J13 (Autodesk Fusion 360 design; units mm, degrees)
part number: 2026-05-31-16-59-09-966
Autodesk Fusion 360 part; units mm, degrees
sketch "Sketch1" plane through (0, 0, 0) normal (0, 0, 1) x (1, 0, 0)
  line L0 (0, 0) -> (40, 0)
  line L1 (40, 0) -> (40, 40)
  line L2 (40, 40) -> (0, 40)
  line L3 (0, 40) -> (0, 0)
  dimension "d1" = 40
  dimension "d2" = 40
  constraint horizontal L0
  constraint vertical L1
  constraint horizontal L2
  constraint vertical L3
  constraint coincident L0.start L3.end
  measures "d1" distance of L0.start L0.end
  measures "d2" distance of L0.start L2.end
extrude "Extrude1" add sketch "Sketch1" along normal blind 5 makes body 1
sketch "Sketch2" plane through (0, 0, 5) normal (0, 0, 1) x (-1, 0, 0)
  line L0 (0, -40) -> (0, 0)
  line L1 (0, 0) -> (-40, 0)
  line L2 (-40, 0) -> (-40, -40)
  line L3 (-40, -40) -> (0, -40)
  line L4 (0, -40) -> (-40, -40)
  line L5 (-40, -40) -> (-40, 0)
  line L6 (-40, 0) -> (0, 0)
  line L7 (0, 0) -> (0, -40)
  line L8 (-38.5, -1.5) -> (-1.5, -1.5)
  line L9 (-1.5, -1.5) -> (-1.5, -38.5)
  line L10 (-1.5, -38.5) -> (-38.5, -38.5)
  line L11 (-38.5, -38.5) -> (-38.5, -1.5)
  constraint horizontal L4
  constraint vertical L5
  constraint horizontal L6
  constraint vertical L7
  constraint coincident L1.end L2.start
  constraint coincident L0.start L3.end
  constraint horizontal L8
  constraint vertical L9
  constraint horizontal L10
  constraint vertical L11
extrude "Extrude2" add sketch "Sketch2" along normal blind 30 bodies 1
sketch "Sketch3" plane through (0, 0, 5) normal (0, 0, 1) x (-1, 0, 0)
  line L0 (-1.5, -38.5) -> (-1.5, -1.5)
  line L1 (-1.5, -1.5) -> (-38.5, -1.5)
  line L2 (-38.5, -1.5) -> (-38.5, -38.5)
  line L3 (-38.5, -38.5) -> (-1.5, -38.5)
  circle A0 centre (-20, -20) radius 15.2
  dimension "d7" = 30.4
  measures "d7" diameter of A0
extrude "Extrude3" cut sketch "Sketch3" against normal blind 49 contours A0 bodies 1
sketch "Sketch4" plane through (0, 0, 0) normal (0, 0, -1) x (1, 0, 0)
  circle A0 centre (20, -20) radius 15.2
  line L0 (0, 0) -> (0, -40)
  line L1 (0, -40) -> (40, -40)
  line L2 (40, -40) -> (40, 0)
  line L3 (40, 0) -> (0, 0)
  circle A1 centre (20, -20) radius 18.2
  dimension "d10" = 3
extrude "Extrude4" add sketch "Sketch4" along normal blind 25 contours A1 bodies 1
sketch "Sketch5" plane through (0, 0, 0) normal (-1, 0, 0) x (0, -1, 0)
  line L0 (-40, 0) -> (0, 0)
  line L1 (0, 0) -> (0, 35)
  line L2 (0, 35) -> (-40, 35)
  line L3 (-40, 35) -> (-40, 0)
  circle A0 centre (-20, -20) radius 1.25
  circle A1 centre (-20, -8) radius 1.25
  dimension "d13" = 2.5
  dimension "d14" = 2.5
  measures "d13" diameter of A0
  measures "d14" diameter of A1
extrude "Extrude5" cut sketch "Sketch5" against normal blind 49 contours A0 | A1 bodies 1
sketch "Sketch6" plane through (0, 0, 0) normal (-1, 0, 0) x (0, -1, 0)
  line L0 (-40, 0) -> (0, 0)
  line L1 (0, 0) -> (0, 35)
  line L2 (0, 35) -> (-40, 35)
  line L3 (-40, 35) -> (-40, 0)
extrude "Extrude6" add sketch "Sketch6" along normal blind 10 bodies 1
sketch "Sketch7" plane through (1.5, 0, 0) normal (1, 0, 0) x (0, 1, 0)
  line L0 (1.5, 5) -> (38.5, 5)
  line L1 (38.5, 5) -> (38.5, 35)
  line L2 (38.5, 35) -> (1.5, 35)
  line L3 (1.5, 35) -> (1.5, 5)
  line L4 (3.5, 7) -> (36.5, 7)
  line L5 (36.5, 7) -> (36.5, 33)
  line L6 (36.5, 33) -> (3.5, 33)
  line L7 (3.5, 33) -> (3.5, 7)
  dimension "d19" = -2
extrude "Extrude7" cut sketch "Sketch7" against normal blind 10 contours L4 L5 L6 L7 bodies 1
fillet "Fillet1" radius 5 1 faces at (-10, 26.6667, 23.3333) on bodies 1
sketch "Sketch8" plane through (38.5, 0, 0) normal (-1, 0, 0) x (0, -1, 0)
  line L0 (-38.5, 5) -> (-1.5, 5)
  line L1 (-1.5, 5) -> (-1.5, 35)
  line L2 (-1.5, 35) -> (-38.5, 35)
  line L3 (-38.5, 35) -> (-38.5, 5)
extrude "Extrude8" cut sketch "Sketch8" against normal blind 7 bodies 1
sketch "Sketch9" plane through (40, 0, 0) normal (1, 0, 0) x (0, 1, 0)
  line L0 (38.5, 35) -> (38.5, 5)
  line L1 (38.5, 5) -> (1.5, 5)
  line L2 (1.5, 5) -> (1.5, 35)
  line L3 (1.5, 35) -> (0, 35)
  line L4 (0, 35) -> (0, 0)
  line L5 (0, 0) -> (40, 0)
  line L6 (40, 0) -> (40, 35)
  line L7 (40, 35) -> (38.5, 35)
  line L8 (0, 35) -> (1.5, 35)
  line L9 (1.5, 35) -> (1.5, 0)
  line L10 (1.5, 0) -> (0, 0)
  line L11 (0, 0) -> (0, 35)
  constraint horizontal L8
  constraint vertical L9
  constraint horizontal L10
  constraint vertical L11
  constraint coincident L5 L9.end
  constraint coincident L3.end L4.start
extrude "Extrude9" add sketch "Sketch9" along normal blind 24 contours L2 L3 L4 L5 L8 L9 L10 L11 bodies 1
sketch "Sketch10" plane through (0, 1.5, 0) normal (0, 1, 0) x (-1, 0, 0)
  line L0 (-40, 5) -> (-1.5, 5)
  line L1 (-1.5, 5) -> (-1.5, 35)
  line L2 (-1.5, 35) -> (-64, 35)
  line L3 (-64, 35) -> (-64, 0)
  line L4 (-64, 0) -> (-40, 0)
  line L5 (-40, 0) -> (-40, 5)
  line L6 (-64, 35) -> (-60, 35)
  line L7 (-60, 35) -> (-60, 0)
  line L8 (-60, 0) -> (-64, 0)
  line L9 (-64, 0) -> (-64, 35)
  constraint horizontal L6
  constraint vertical L7
  constraint horizontal L8
  constraint vertical L9
  constraint coincident L4 L7.end
  constraint coincident L2.end L3.start
extrude "Extrude10" add sketch "Sketch10" along normal blind 40 contours L2 L3 L4 L6 L7 L8 L9 bodies 1
sketch "Sketch11" plane through (60, 0, 0) normal (-1, 0, 0) x (0, -1, 0)
  line L0 (-1.5, 0) -> (-1.5, 35)
  line L1 (-1.5, 35) -> (-41.5, 35)
  line L2 (-41.5, 35) -> (-41.5, 0)
  line L3 (-41.5, 0) -> (-1.5, 0)
  line L4 (-41.5, 35) -> (-35, 35)
  line L5 (-35, 35) -> (-35, 0)
  line L6 (-35, 0) -> (-41.5, 0)
  line L7 (-41.5, 0) -> (-41.5, 35)
  constraint horizontal L4
  constraint vertical L5
  constraint horizontal L6
  constraint vertical L7
  constraint coincident L3 L5.end
  constraint coincident L1.end L2.start
extrude "Extrude11" add sketch "Sketch11" along normal blind 7 contours L1 L2 L3 L4 L5 L6 L7 bodies 1
sketch "Sketch12" plane through (40, 0, 0) normal (1, 0, 0) x (0, 1, 0)
  line L0 (1.5, 5) -> (1.5, 0)
  line L1 (1.5, 0) -> (40, 0)
  line L2 (40, 0) -> (40, 35)
  line L3 (40, 35) -> (38.5, 35)
  line L4 (38.5, 35) -> (38.5, 5)
  line L5 (38.5, 5) -> (1.5, 5)
  line L6 (38.5, 35) -> (40, 35)
  line L7 (40, 35) -> (40, 0)
  line L8 (40, 0) -> (38.5, 0)
  line L9 (38.5, 0) -> (38.5, 35)
  constraint horizontal L6
  constraint vertical L7
  constraint horizontal L8
  constraint vertical L9
  constraint coincident L1.end L2.start
  constraint coincident L3.end L4.start
extrude "Extrude12" add sketch "Sketch12" along normal blind 13 contours L1 L2 L3 L4 L6 L7 L8 L9 bodies 1
fillet "Fillet2" radius 17 1 edges at (64, 41.5, 17.5) on bodies 1
sketch "Sketch13" plane through (0, 40, 0) normal (0, 1, 0) x (-1, 0, 0)
  line L0 (5, 0) -> (5, 35)
  line L1 (5, 35) -> (-53, 35)
  line L2 (-53, 35) -> (-53, 0)
  line L3 (-53, 0) -> (5, 0)
  line L4 (-24.9639, 7.5563) -> (-6.6598, 7.5563)
  line L5 (-6.6598, 7.5563) -> (-6.6598, 25)
  line L6 (-16.6598, 35) -> (-34.9639, 35)
  line L7 (-34.9639, 35) -> (-34.9639, 17.5563)
  arc A0 (-34.9639, 17.5563) -> (-24.9639, 7.5563) centre (-24.9639, 17.5563) ccw
  arc A1 (-6.6598, 25) -> (-16.6598, 35) centre (-16.6598, 25) ccw
  dimension "d36" = 10
  constraint horizontal L4
  constraint vertical L5
  constraint horizontal L6
  constraint vertical L7
  constraint tangent L4 A0
  constraint tangent L7 A0
  constraint tangent L5 A1
  constraint tangent L6 A1
  constraint equal A0 A1
  measures "d36" radius of A0
extrude "Extrude13" cut sketch "Sketch13" against normal blind 10 contours L1 L4 L5 L6 L7 A0 A1 bodies 1
sketch "Sketch14" plane through (0, 40, 0) normal (0, 1, 0) x (-1, 0, 0)
  arc A0 (-6.6598, 25) -> (-16.6598, 35) centre (-16.6598, 25) ccw
  line L0 (-6.6598, 25) -> (-6.6598, 7.5563)
  line L1 (-6.6598, 7.5563) -> (-24.9639, 7.5563)
  arc A1 (-34.9639, 17.5563) -> (-24.9639, 7.5563) centre (-24.9639, 17.5563) ccw
  line L2 (-34.9639, 17.5563) -> (-34.9639, 35)
  line L3 (-34.9639, 35) -> (-53, 35)
  line L4 (-53, 35) -> (-53, 0)
  line L5 (-53, 0) -> (5, 0)
  line L6 (5, 0) -> (5, 35)
  line L7 (5, 35) -> (-16.6598, 35)
  line L8 (-34.9639, 35) -> (-15, 35)
  constraint coincident L2.end L3.start
  constraint coincident L7 L8.end
extrude "Extrude14" add sketch "Sketch14" along normal blind 10 separate body contours A0 L0 L1 A1 L2 L8 makes body 2
fillet "Fillet3" radius 4.5 1 faces at (25.5292, 50, 20.0375) on bodies 2
sketch "Sketch15" plane through (0, 50, 0) normal (0, 1, 0) x (-1, 0, 0)
  line L0 (-30.4639, 30.5) -> (-30.4639, 17.5563)
  arc A0 (-30.4639, 17.5563) -> (-24.9639, 12.0563) centre (-24.9639, 17.5563) ccw
  line L1 (-24.9639, 12.0563) -> (-11.1598, 12.0563)
  line L2 (-11.1598, 12.0563) -> (-11.1598, 25)
  arc A1 (-11.1598, 25) -> (-16.6598, 30.5) centre (-16.6598, 25) ccw
  line L3 (-16.6598, 30.5) -> (-30.4639, 30.5)
sketch "Sketch16" plane through (0, 50, 0) normal (0, 1, 0) x (-1, 0, 0)
  circle A0 centre (-20, 21) radius 5
  circle A1 centre (-20, 21) radius 6
  dimension "d43" = 1
extrude "Extrude15" add sketch "Sketch16" along normal blind 3 bodies 2
sketch "Sketch17" plane through (0, 50, 0) normal (0, 1, 0) x (-1, 0, 0)
  circle A0 centre (-20, 21) radius 4.8253
extrude "Extrude16" cut sketch "Sketch17" against normal blind 25 bodies 2
sketch "Sketch18" plane through (0, 40, 0) normal (0, -1, 0) x (1, 0, 0)
  circle A0 centre (20, 21) radius 4.8253
  arc A1 (24.9639, 7.5563) -> (34.9639, 17.5563) centre (24.9639, 17.5563) ccw
  line L0 (34.9639, 17.5563) -> (34.9639, 35)
  line L1 (34.9639, 35) -> (16.6598, 35)
  arc A2 (16.6598, 35) -> (6.6598, 25) centre (16.6598, 25) ccw
  line L2 (6.6598, 25) -> (6.6598, 7.5563)
  line L3 (6.6598, 7.5563) -> (24.9639, 7.5563)
  line L4 (7.3732, 25) -> (7.3732, 8.2697)
  line L5 (7.3732, 8.2697) -> (24.9639, 8.2697)
  arc A3 (24.9639, 8.2697) -> (34.2505, 17.5563) centre (24.9639, 17.5563) ccw
  line L6 (34.2505, 17.5563) -> (34.2505, 34.2866)
  line L7 (34.2505, 34.2866) -> (16.6598, 34.2866)
  arc A4 (16.6598, 34.2866) -> (7.3732, 25) centre (16.6598, 25) ccw
  dimension "d48" = -0.7134
extrude "Extrude17" cut sketch "Sketch18" against normal blind 7 contours L4 L5 A3 L6 L7 A4 bodies 2
extrude "Extrude18" cut 1 faces at (-2.8333, 13.8333, 35) along direction (0, 0, -1) blind 5 on bodies 1 bodies 1
extrude "Extrude19" cut 1 faces at (-5, 1.1667, 32.6667) along direction (-1, 0, 0) blind 7 on bodies 1 bodies 1
sketch "Sketch19" plane through (-8.5, 0, 0) normal (1, 0, 0) x (0, 1, 0)
  line L0 (3.5, 30) -> (3.5, 7)
  line L1 (3.5, 7) -> (36.5, 7)
  line L2 (36.5, 7) -> (36.5, 30)
  line L3 (36.5, 30) -> (36.5, 33)
  line L4 (36.5, 33) -> (3.5, 33)
  line L5 (3.5, 33) -> (3.5, 30)
